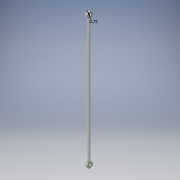
# Autodesk Inventor part: longbar
Saved by Autodesk Inventor 2016 (Build 200138000, 138)
## iProperties
Created: 2016-04-21
Part Number: longbar
Material: Generic
Document SubType Name: Modeling
Designer: Sam
Density: 1 g/cm^3
Appearance: Default
Author: Sam
Autodesk Inventor part; units mm, degrees
ref_plane "YZ Plane" through (0, 0, 0) normal (1, 0, 0) x (0, 1, 0)
ref_plane "XZ Plane" through (0, 0, 0) normal (0, 1, 0) x (-1, 0, 0)
ref_plane "XY Plane" through (0, 0, 0) normal (0, 0, 1) x (1, 0, 0)
sketch "Sketch1" plane through (0, 0, 0) normal (1, 0, 0) x (0, 1, 0)
  point P0 (0, 0)
sketch "Sketch2" plane through (0, 0, 0) normal (0, 1, 0) x (-1, 0, 0)
  circle A0 centre (0, 0) radius 1.5
  dimension "d0" = 3
  constraints: 1 centre point, 1 coincident
  measures "d0" diameter of A0
extrude "Extrusion1" add sketch "Sketch2" along normal mid plane 170
sketch "Sketch3" plane through (0, 0, 0) normal (0, 0, 1) x (1, 0, 0)
  line L0 (1.5, 85) -> (-1.5, 85) projected
  arc A0 (-2.5, 87.5) -> (1.5, 85.5) centre (0, 87.5) ccw
  arc A1 (-3.75, 87.5) -> (1.5, 84.0631) centre (0, 87.5) ccw
  line L1 (1.5, 84.0631) -> (1.5, 85.5)
  line L2 (-2.5, 87.5) -> (-3.75, 87.5)
  line L3 (0, 87.5) -> (4.1351, 87.5) construction
  line L4 (1.5, -85) -> (-1.5, -85)
  arc A2 (1.5, -85.5) -> (-2.5, -87.5) centre (0, -87.5) ccw
  arc A3 (1.5, -84.0631) -> (-3.75, -87.5) centre (0, -87.5) ccw
  line L5 (1.5, -84.0631) -> (1.5, -85.5)
  line L6 (-2.5, -87.5) -> (-3.75, -87.5)
  line L7 (0, -87.5) -> (4.1351, -87.5) construction
  dimension "d4" = 7.5
  constraints: 14 end point, 8 point on circle, 4 centre point, 2 coincident, 2 horizontal, 1 vertical
  measures "d4" diameter of A1
revolve "Revolution1" add sketch "Sketch3" angle 360 about axis through (0, 87.5, 0) along (1, 0, 0) contours L1 A1 L2 A0 L0 | L0 A0 L1
revolve "Revolution2" add sketch "Sketch3" angle 360 about axis through (0, -87.5, 0) along (1, 0, 0) contours L5 A2 L4 | L4 A2 L6 A3 L5
body "Solid1"
